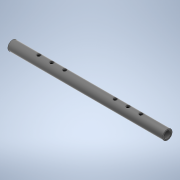
# Autodesk Inventor part: cross-beam
Saved by Autodesk Inventor 2022 (Build 260153000, 153)
## iProperties
Created: 2021-12-05
Part Number: cross-beam
Material: Generic
Document SubType Name: Modeling
Designer: Vedic
Density: 1 g/cm^3
Appearance: Default
Author: Vedic
Autodesk Inventor part; units mm, degrees
ref_plane "YZ Plane" through (0, 0, 0) normal (1, 0, 0) x (0, 1, 0)
ref_plane "XY Plane" through (0, 0, 0) normal (0, 0, 1) x (1, 0, 0)
sketch "Sketch1" plane through (0, 0, 0) normal (1, 0, 0) x (0, 1, 0)
  circle A0 centre (0, 0) radius 9.525
  circle A1 centre (0, 0) radius 6.985
  dimension "d0" = 19.05
  dimension "d1" = 2.54
  constraints: 2 centre point, 1 coincident
  measures "d0" diameter of A0
  measures "d1" radial gap between concentric circles of A0 A1
extrude "Extrusion1" add sketch "Sketch1" along normal blind 304.8
ref_plane "Work Plane1" through (0, 14.2875, 0) normal (0, 1, 0) x (-1, 0, 0)
sketch "Sketch2" plane through (0, 14.2875, 0) normal (0, 1, 0) x (-1, 0, 0)
  line L0 (0, 0) -> (-304.8, 0) construction
  line L1 (-304.8, 9.525) -> (-304.8, -9.525) projected
  circle A0 centre (-51.9303, 0) radius 3.175
  circle A1 centre (-77.3303, 0) radius 3.175
  circle A2 centre (-227.4697, 0) radius 3.175
  circle A3 centre (-252.8697, 0) radius 3.175
  line L2 (0, -9.525) -> (-304.8, -9.525) projected
  line L3 (-152.4, -9.525) -> (-152.4, 9.525)
  line L4 (0, 9.525) -> (-304.8, 9.525) projected
  circle A4 centre (-102.7303, 0) radius 3.175
  circle A5 centre (-202.0697, 0) radius 3.175
  dimension "d5" = 6.35
  dimension "d9" = 25.4
  dimension "d10" = 25.4
  dimension "d17" = 25.4
  dimension "d18" = 25.4
  dimension "d19" = 150.1394
  dimension "d20" = 75.0697
  constraints: 6 centre point, 6 point on line, 5 equal radius, 4 end point, 3 midpoint
  measures "d5" diameter of A0
  measures "d9" distance of A1.centre A0.centre
  measures "d10" distance of A3.centre A2.centre
  measures "d17" distance of A2.centre A5.centre
  measures "d18" distance of A4.centre A1.centre
  measures "d19" distance of A2.centre A1.centre
  measures "d20" distance from line of L3 A1.centre
extrude "Extrusion2" cut sketch "Sketch2" against normal through all contours A0 | A1 | A2 | A3 | A4 | A5
equation "\"d18\" = d9"
equation "\"d20\" = 0.5 * d19"
body "Solid1"
